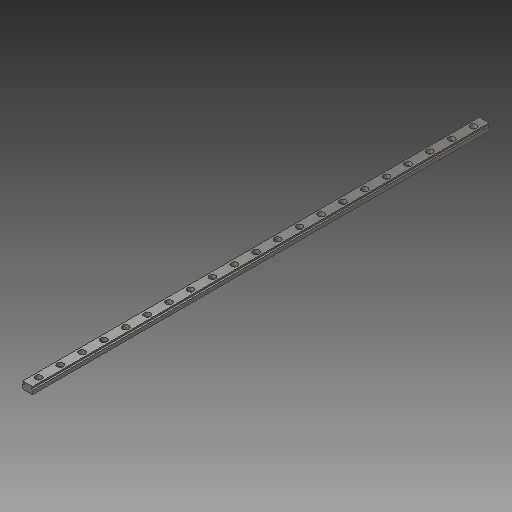
# Autodesk Inventor part: MGN-9 Rail 470mm
Saved by Autodesk Inventor 2019 (Build 230136000, 136)
## iProperties
Created: 2018-10-13
Part Number: MGN-9 Rail 470mm
Material: Stainless Steel
Document SubType Name: Modeling
Designer: Ax
Density: 8 g/cm^3
Appearance: Semi-Polished
Mass: 163.972 g
Surface Area: 163.096 cm^2
Volume: 20.4965 cm^3
Author: Ax
Autodesk Inventor part; units mm, degrees
ref_plane "YZ Plane" through (0, 0, 0) normal (1, 0, 0) x (0, 1, 0)
ref_plane "XZ Plane" through (0, 0, 0) normal (0, 1, 0) x (-1, 0, 0)
ref_plane "XY Plane" through (0, 0, 0) normal (0, 0, 1) x (1, 0, 0)
sketch "Sketch1" plane through (0, 0, 0) normal (0, 0, 1) x (1, 0, 0)
  line L0 (-4.5, -3.25) -> (4.5, -3.25)
  line L1 (4.5, 3.25) -> (-4.5, 3.25)
  line L2 (-4.5, -3.25) -> (4.5, 3.25) construction
  line L3 (4.5, -3.25) -> (-4.5, 3.25) construction
  line L4 (-4.5, 1.25) -> (4.5, 1.25) construction
  line L5 (-3.564, 1.602) -> (-3.235, 1.602)
  line L6 (-3.235, 1.602) -> (-3.235, 0.898)
  line L7 (-3.235, 0.898) -> (-3.564, 0.898)
  arc A0 (-4.5, 0.25) -> (-3.564, 0.898) centre (-4.5, 1.25) ccw
  arc A1 (-3.564, 1.602) -> (-4.5, 2.25) centre (-4.5, 1.25) ccw
  line L8 (0, 3.25) -> (0, -3.25) construction
  line L9 (3.564, 1.602) -> (3.235, 1.602)
  line L10 (3.235, 1.602) -> (3.235, 0.898)
  line L11 (3.235, 0.898) -> (3.564, 0.898)
  arc A2 (3.564, 0.898) -> (4.5, 0.25) centre (4.5, 1.25) ccw
  arc A3 (4.5, 2.25) -> (3.564, 1.602) centre (4.5, 1.25) ccw
  line L12 (-4.5, 3.25) -> (-4.5, 2.25)
  line L13 (-4.5, 0.25) -> (-4.5, -3.25)
  line L14 (4.5, -3.25) -> (4.5, 0.25)
  line L15 (4.5, 2.25) -> (4.5, 3.25)
  line L16 (4.5, 2.25) -> (4.5, 0.25) construction
  line L17 (-4.5, 2.25) -> (-4.5, 0.25) construction
  point P0 (0, 0)
  dimension "d0" = 9
  dimension "d1" = 6.5
  dimension "d3" = 2
  dimension "d4" = 1
  dimension "d5" = 0.329
  dimension "d6" = 0.704
  constraints: 36 end point, 8 point on circle, 7 symmetric about line, 6 perpendicular, 5 midpoint, 5 parallel, 4 centre point, 2 horizontal, 2 vertical, 1 concentric, 2 other
  measures "d0" distance of L1.end L1.start
  measures "d1" distance of L0.end L1.start
  measures "d3" distance of L1.end L4.start
  measures "d4" radius of A0
  measures "d5" distance of L6.end L7.end
  measures "d6" distance of L5.end L6.end
extrude "Extrusion1" add sketch "Sketch1" along normal mid plane 420
sketch "Sketch2" plane through (-4.5, 3.25, 210) normal (0, 1, 0) x (1, 0, 0)
  circle A0 centre (4.5, 210) radius 1.6
  dimension "d9" = 3.2
  constraints: 1 centre point, 1 coincident
  measures "d9" diameter of A0
extrude "Extrusion2" cut sketch "Sketch2" against normal through all
pattern_linear "Rectangular Pattern1" count 23 spacing 20 along (0, 0, 1) of "Extrusion2" first direction both ways yes
sketch "Sketch3" plane through (-4.5, 3.25, 210) normal (0, 1, 0) x (1, 0, 0)
  circle A0 centre (4.5, 210) radius 3
  dimension "d15" = 6
  constraints: 1 centre point, 1 coincident
  measures "d15" diameter of A0
extrude "Extrusion3" cut sketch "Sketch3" against normal blind 3.5
pattern_linear "Rectangular Pattern2" count 23 spacing 20 along (0, 0, 1) of "Extrusion3" first direction both ways yes
body "Solid1"
